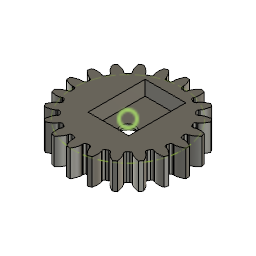
Servo_Gear (Autodesk Fusion 360 archive; units mm, degrees)
design "Servo_Gear"
description: Spur Gear; Module: 1.0; Num Teeth: 20; Pressure Angle: 20.0; Backlash: 0.00 mm
part number: 2026-08-10-18-01-22-383
Autodesk Fusion 360 part; units mm, degrees
(part 1 of 4)
sketch "Base Circle" plane through (0, 0, 0) normal (0, 0, 1) x (1, 0, 0)
  circle A0 centre (0, 0) radius 8.843
  circle A1 centre (0, 0) radius 2.6
  dimension "d9" = 5.2
  measures "d9" diameter of A1
extrude "Extrude1" add sketch "Base Circle" along normal blind 3.5
sketch "Gear Tooth" plane through (0, 0, 0) normal (0, 0, 1) x (1, 0, 0)
  spline S0 degree 5 poles (9.3559, -0.8768) (9.3606, -0.8772) (9.3699, -0.878) (9.3839, -0.8788) (9.4026, -0.8791) (9.426, -0.8785) (9.4495, -0.8772) (9.473, -0.8755) (9.4965, -0.8735) (9.52, -0.8714) (9.5435, -0.8691) (9.567, -0.8666) (9.5906, -0.8638) (9.6142, -0.8607) (9.6377, -0.8572) (9.6613, -0.8535) (9.6849, -0.8494) (9.7085, -0.8451) (9.7321, -0.8406) (9.7557, -0.836) (9.7793, -0.8311) (9.8029, -0.8261) (9.8265, -0.8208) (9.8501, -0.8153) (9.8737, -0.8096) (9.8973, -0.8037) (9.9209, -0.7977) (9.9445, -0.7914) (9.968, -0.7849) (9.9916, -0.7783) (10.0152, -0.7715) (10.0388, -0.7645) (10.0623, -0.7574) (10.0859, -0.7501) (10.1095, -0.7426) (10.133, -0.7349) (10.1565, -0.7271) (10.1801, -0.7191) (10.2036, -0.711) (10.2271, -0.7027) (10.2506, -0.6942) (10.2741, -0.6856) (10.2976, -0.6768) (10.321, -0.6679) (10.3445, -0.6588) (10.3679, -0.6496) (10.3913, -0.6402) (10.4148, -0.6307) (10.4382, -0.621) (10.4615, -0.6112) (10.4849, -0.6013) (10.5083, -0.5912) (10.5316, -0.5809) (10.5549, -0.5705) (10.5782, -0.56) (10.6015, -0.5493) (10.6248, -0.5385) (10.6481, -0.5276) (10.6713, -0.5165) (10.6945, -0.5053) (10.7177, -0.4939) (10.7409, -0.4824) (10.7641, -0.4708) (10.7872, -0.4591) (10.8103, -0.4472) (10.8334, -0.4352) (10.8565, -0.423) (10.8796, -0.4107) (10.9026, -0.3983) (10.9256, -0.3858) (10.9486, -0.3731) (10.967, -0.3629) (10.9807, -0.3552) (10.9899, -0.35) (10.9945, -0.3474) knots 0 0 0 0 0 0 0.01428571 0.02857143 0.04285714 0.05714286 0.07142857 0.08571429 0.1 0.11428571 0.12857143 0.14285714 0.15714286 0.17142857 0.18571429 0.2 0.21428571 0.22857143 0.24285714 0.25714286 0.27142857 0.28571429 0.3 0.31428571 0.32857143 0.34285714 0.35714286 0.37142857 0.38571429 0.4 0.41428571 0.42857143 0.44285714 0.45714286 0.47142857 0.48571429 0.5 0.51428571 0.52857143 0.54285714 0.55714286 0.57142857 0.58571429 0.6 0.61428571 0.62857143 0.64285714 0.65714286 0.67142857 0.68571429 0.7 0.71428571 0.72857143 0.74285714 0.75714286 0.77142857 0.78571429 0.8 0.81428571 0.82857143 0.84285714 0.85714286 0.87142857 0.88571429 0.9 0.91428571 0.92857143 0.94285714 0.95714286 0.97142857 0.98571429 1 1 1 1 1 1
  spline S1 degree 5 poles (9.3559, 0.8768) (9.3606, 0.8772) (9.3699, 0.878) (9.3839, 0.8788) (9.4026, 0.8791) (9.426, 0.8785) (9.4495, 0.8772) (9.473, 0.8755) (9.4965, 0.8735) (9.52, 0.8714) (9.5435, 0.8691) (9.567, 0.8666) (9.5906, 0.8638) (9.6142, 0.8607) (9.6377, 0.8572) (9.6613, 0.8535) (9.6849, 0.8494) (9.7085, 0.8451) (9.7321, 0.8406) (9.7557, 0.836) (9.7793, 0.8311) (9.8029, 0.8261) (9.8265, 0.8208) (9.8501, 0.8153) (9.8737, 0.8096) (9.8973, 0.8037) (9.9209, 0.7977) (9.9445, 0.7914) (9.968, 0.7849) (9.9916, 0.7783) (10.0152, 0.7715) (10.0388, 0.7645) (10.0623, 0.7574) (10.0859, 0.7501) (10.1095, 0.7426) (10.133, 0.7349) (10.1565, 0.7271) (10.1801, 0.7191) (10.2036, 0.711) (10.2271, 0.7027) (10.2506, 0.6942) (10.2741, 0.6856) (10.2976, 0.6768) (10.321, 0.6679) (10.3445, 0.6588) (10.3679, 0.6496) (10.3913, 0.6402) (10.4148, 0.6307) (10.4382, 0.621) (10.4615, 0.6112) (10.4849, 0.6013) (10.5083, 0.5912) (10.5316, 0.5809) (10.5549, 0.5705) (10.5782, 0.56) (10.6015, 0.5493) (10.6248, 0.5385) (10.6481, 0.5276) (10.6713, 0.5165) (10.6945, 0.5053) (10.7177, 0.4939) (10.7409, 0.4824) (10.7641, 0.4708) (10.7872, 0.4591) (10.8103, 0.4472) (10.8334, 0.4352) (10.8565, 0.423) (10.8796, 0.4107) (10.9026, 0.3983) (10.9256, 0.3858) (10.9486, 0.3731) (10.967, 0.3629) (10.9807, 0.3552) (10.9899, 0.35) (10.9945, 0.3474) knots 0 0 0 0 0 0 0.01428571 0.02857143 0.04285714 0.05714286 0.07142857 0.08571429 0.1 0.11428571 0.12857143 0.14285714 0.15714286 0.17142857 0.18571429 0.2 0.21428571 0.22857143 0.24285714 0.25714286 0.27142857 0.28571429 0.3 0.31428571 0.32857143 0.34285714 0.35714286 0.37142857 0.38571429 0.4 0.41428571 0.42857143 0.44285714 0.45714286 0.47142857 0.48571429 0.5 0.51428571 0.52857143 0.54285714 0.55714286 0.57142857 0.58571429 0.6 0.61428571 0.62857143 0.64285714 0.65714286 0.67142857 0.68571429 0.7 0.71428571 0.72857143 0.74285714 0.75714286 0.77142857 0.78571429 0.8 0.81428571 0.82857143 0.84285714 0.85714286 0.87142857 0.88571429 0.9 0.91428571 0.92857143 0.94285714 0.95714286 0.97142857 0.98571429 1 1 1 1 1 1
  arc A0 (10.9945, -0.3474) -> (10.9945, 0.3474) centre (0, 0) ccw
  line L0 (8.7945, -0.8242) -> (9.3559, -0.8768)
  line L1 (8.7945, 0.8242) -> (9.3559, 0.8768)
  line L2 (8.7945, -0.8242) -> (8.7945, 0.8242)
  point P0 (9.471, -0.8756)
  point P1 (9.5871, -0.8642)
  point P2 (9.7036, -0.846)
  point P3 (9.8206, -0.8221)
  point P4 (9.9379, -0.7931)
  point P5 (10.0553, -0.7595)
  point P6 (10.1729, -0.7215)
  point P7 (10.2906, -0.6794)
  point P8 (10.4082, -0.6333)
  point P9 (10.5258, -0.5834)
  point P10 (10.6433, -0.5298)
  point P11 (10.7606, -0.4725)
  point P12 (10.8777, -0.4117)
  point P13 (9.471, 0.8756)
  point P14 (9.5871, 0.8642)
  point P15 (9.7036, 0.846)
  point P16 (9.8206, 0.8221)
  point P17 (9.9379, 0.7931)
  point P18 (10.0553, 0.7595)
  point P19 (10.1729, 0.7215)
  point P20 (10.2906, 0.6794)
  point P21 (10.4082, 0.6333)
  point P22 (10.5258, 0.5834)
  point P23 (10.6433, 0.5298)
  point P24 (10.7606, 0.4725)
  point P25 (10.8777, 0.4117)
extrude "Extrude2" add sketch "Gear Tooth" along normal blind 3.5
fillet "Fillet1" radius 0.35 2 edges at (8.8044, -0.8251, 1.75) (8.8044, 0.8251, 1.75)
pattern_circular "C-Pattern1" count 20 over 360 about axis through (0, 0, 0) along (0, 0, 1) of "Extrude2", "Fillet1"
sketch "Diametrial Pitch Circle" plane through (0, 0, 0) normal (0, 0, 1) x (1, 0, 0)
  circle A0 centre (0, 0) radius 10 construction
extrude "Extrude3" add 1 faces at (6.7196, 0, 3.5) along direction (0, 0, 1) blind 0.4
sketch "Sketch4" plane through (0, 0, 3.9) normal (0, 0, 1) x (-1, 0, 0)
  arc A0 (-8.6959, 1.6061) -> (-8.7666, 1.1597) centre (0, 0) ccw
  arc A1 (-9.1463, 0.8572) -> (-8.7666, 1.1597) centre (-9.1136, 1.2056) ccw
  line L0 (-9.1463, 0.8572) -> (-9.3559, 0.8768)
  spline S0 degree 5 poles (-9.3559, 0.8768) (-9.3606, 0.8772) (-9.3699, 0.878) (-9.3839, 0.8788) (-9.4026, 0.8791) (-9.426, 0.8785) (-9.4495, 0.8772) (-9.473, 0.8755) (-9.4965, 0.8735) (-9.52, 0.8714) (-9.5435, 0.8691) (-9.567, 0.8666) (-9.5906, 0.8638) (-9.6142, 0.8607) (-9.6377, 0.8572) (-9.6613, 0.8535) (-9.6849, 0.8494) (-9.7085, 0.8451) (-9.7321, 0.8406) (-9.7557, 0.836) (-9.7793, 0.8311) (-9.8029, 0.8261) (-9.8265, 0.8208) (-9.8501, 0.8153) (-9.8737, 0.8096) (-9.8973, 0.8037) (-9.9209, 0.7977) (-9.9445, 0.7914) (-9.968, 0.7849) (-9.9916, 0.7783) (-10.0152, 0.7715) (-10.0388, 0.7645) (-10.0623, 0.7574) (-10.0859, 0.7501) (-10.1095, 0.7426) (-10.133, 0.7349) (-10.1565, 0.7271) (-10.1801, 0.7191) (-10.2036, 0.711) (-10.2271, 0.7027) (-10.2506, 0.6942) (-10.2741, 0.6856) (-10.2976, 0.6768) (-10.321, 0.6679) (-10.3445, 0.6588) (-10.3679, 0.6496) (-10.3913, 0.6402) (-10.4148, 0.6307) (-10.4382, 0.621) (-10.4615, 0.6112) (-10.4849, 0.6013) (-10.5083, 0.5912) (-10.5316, 0.5809) (-10.5549, 0.5705) (-10.5782, 0.56) (-10.6015, 0.5493) (-10.6248, 0.5385) (-10.6481, 0.5276) (-10.6713, 0.5165) (-10.6945, 0.5053) (-10.7177, 0.4939) (-10.7409, 0.4824) (-10.7641, 0.4708) (-10.7872, 0.4591) (-10.8103, 0.4472) (-10.8334, 0.4352) (-10.8565, 0.423) (-10.8796, 0.4107) (-10.9026, 0.3983) (-10.9256, 0.3858) (-10.9486, 0.3731) (-10.967, 0.3629) (-10.9807, 0.3552) (-10.9899, 0.35) (-10.9945, 0.3474) knots 0 0 0 0 0 0 0.01428571 0.02857143 0.04285714 0.05714286 0.07142857 0.08571429 0.1 0.11428571 0.12857143 0.14285714 0.15714286 0.17142857 0.18571429 0.2 0.21428571 0.22857143 0.24285714 0.25714286 0.27142857 0.28571429 0.3 0.31428571 0.32857143 0.34285714 0.35714286 0.37142857 0.38571429 0.4 0.41428571 0.42857143 0.44285714 0.45714286 0.47142857 0.48571429 0.5 0.51428571 0.52857143 0.54285714 0.55714286 0.57142857 0.58571429 0.6 0.61428571 0.62857143 0.64285714 0.65714286 0.67142857 0.68571429 0.7 0.71428571 0.72857143 0.74285714 0.75714286 0.77142857 0.78571429 0.8 0.81428571 0.82857143 0.84285714 0.85714286 0.87142857 0.88571429 0.9 0.91428571 0.92857143 0.94285714 0.95714286 0.97142857 0.98571429 1 1 1 1 1 1
  arc A2 (-10.9945, 0.3474) -> (-10.9945, -0.3474) centre (0, 0) ccw
  spline S1 degree 5 poles (-10.9945, -0.3474) (-10.9899, -0.35) (-10.9807, -0.3552) (-10.967, -0.3629) (-10.9486, -0.3731) (-10.9256, -0.3858) (-10.9026, -0.3983) (-10.8796, -0.4107) (-10.8565, -0.423) (-10.8334, -0.4352) (-10.8103, -0.4472) (-10.7872, -0.4591) (-10.7641, -0.4708) (-10.7409, -0.4824) (-10.7177, -0.4939) (-10.6945, -0.5053) (-10.6713, -0.5165) (-10.6481, -0.5276) (-10.6248, -0.5385) (-10.6015, -0.5493) (-10.5782, -0.56) (-10.5549, -0.5705) (-10.5316, -0.5809) (-10.5083, -0.5912) (-10.4849, -0.6013) (-10.4615, -0.6112) (-10.4382, -0.621) (-10.4148, -0.6307) (-10.3913, -0.6402) (-10.3679, -0.6496) (-10.3445, -0.6588) (-10.321, -0.6679) (-10.2976, -0.6768) (-10.2741, -0.6856) (-10.2506, -0.6942) (-10.2271, -0.7027) (-10.2036, -0.711) (-10.1801, -0.7191) (-10.1565, -0.7271) (-10.133, -0.7349) (-10.1095, -0.7426) (-10.0859, -0.7501) (-10.0623, -0.7574) (-10.0388, -0.7645) (-10.0152, -0.7715) (-9.9916, -0.7783) (-9.968, -0.7849) (-9.9445, -0.7914) (-9.9209, -0.7977) (-9.8973, -0.8037) (-9.8737, -0.8096) (-9.8501, -0.8153) (-9.8265, -0.8208) (-9.8029, -0.8261) (-9.7793, -0.8311) (-9.7557, -0.836) (-9.7321, -0.8406) (-9.7085, -0.8451) (-9.6849, -0.8494) (-9.6613, -0.8535) (-9.6377, -0.8572) (-9.6142, -0.8607) (-9.5906, -0.8638) (-9.567, -0.8666) (-9.5435, -0.8691) (-9.52, -0.8714) (-9.4965, -0.8735) (-9.473, -0.8755) (-9.4495, -0.8772) (-9.426, -0.8785) (-9.4026, -0.8791) (-9.3839, -0.8788) (-9.3699, -0.878) (-9.3606, -0.8772) (-9.3559, -0.8768) knots -1 -1 -1 -1 -1 -1 -0.98571429 -0.97142857 -0.95714286 -0.94285714 -0.92857143 -0.91428571 -0.9 -0.88571429 -0.87142857 -0.85714286 -0.84285714 -0.82857143 -0.81428571 -0.8 -0.78571429 -0.77142857 -0.75714286 -0.74285714 -0.72857143 -0.71428571 -0.7 -0.68571429 -0.67142857 -0.65714286 -0.64285714 -0.62857143 -0.61428571 -0.6 -0.58571429 -0.57142857 -0.55714286 -0.54285714 -0.52857143 -0.51428571 -0.5 -0.48571429 -0.47142857 -0.45714286 -0.44285714 -0.42857143 -0.41428571 -0.4 -0.38571429 -0.37142857 -0.35714286 -0.34285714 -0.32857143 -0.31428571 -0.3 -0.28571429 -0.27142857 -0.25714286 -0.24285714 -0.22857143 -0.21428571 -0.2 -0.18571429 -0.17142857 -0.15714286 -0.14285714 -0.12857143 -0.11428571 -0.1 -0.08571429 -0.07142857 -0.05714286 -0.04285714 -0.02857143 -0.01428571 0 0 0 0 0 0
  line L1 (-9.3559, -0.8768) -> (-9.1463, -0.8572)
  arc A3 (-8.7666, -1.1597) -> (-9.1463, -0.8572) centre (-9.1136, -1.2056) ccw
  arc A4 (-8.7666, -1.1597) -> (-8.6959, -1.6061) centre (0, 0) ccw
  arc A5 (-8.9635, -2.0111) -> (-8.6959, -1.6061) centre (-9.0401, -1.6696) ccw
  line L2 (-8.9635, -2.0111) -> (-9.169, -2.0572)
  spline S2 degree 5 poles (-9.169, -2.0572) (-9.1735, -2.0583) (-9.1826, -2.0604) (-9.1962, -2.064) (-9.2141, -2.0695) (-9.2361, -2.0773) (-9.2581, -2.0858) (-9.2799, -2.0947) (-9.3016, -2.1038) (-9.3233, -2.1131) (-9.345, -2.1225) (-9.3666, -2.1322) (-9.3881, -2.1421) (-9.4096, -2.1524) (-9.4309, -2.1629) (-9.4522, -2.1738) (-9.4734, -2.185) (-9.4945, -2.1963) (-9.5155, -2.2079) (-9.5365, -2.2196) (-9.5575, -2.2315) (-9.5784, -2.2436) (-9.5992, -2.2559) (-9.6199, -2.2684) (-9.6406, -2.2811) (-9.6612, -2.294) (-9.6818, -2.3071) (-9.7023, -2.3204) (-9.7227, -2.3338) (-9.7431, -2.3474) (-9.7634, -2.3611) (-9.7837, -2.375) (-9.8039, -2.3891) (-9.8241, -2.4033) (-9.8441, -2.4177) (-9.8642, -2.4323) (-9.8841, -2.447) (-9.904, -2.4619) (-9.9239, -2.4769) (-9.9437, -2.492) (-9.9634, -2.5074) (-9.9831, -2.5228) (-10.0027, -2.5384) (-10.0223, -2.5541) (-10.0418, -2.57) (-10.0612, -2.586) (-10.0806, -2.6022) (-10.0999, -2.6185) (-10.1192, -2.6349) (-10.1384, -2.6515) (-10.1575, -2.6682) (-10.1766, -2.685) (-10.1957, -2.702) (-10.2146, -2.719) (-10.2335, -2.7363) (-10.2524, -2.7536) (-10.2712, -2.7711) (-10.2899, -2.7887) (-10.3086, -2.8064) (-10.3272, -2.8242) (-10.3458, -2.8422) (-10.3643, -2.8603) (-10.3827, -2.8785) (-10.4011, -2.8968) (-10.4194, -2.9153) (-10.4377, -2.9339) (-10.4559, -2.9525) (-10.474, -2.9713) (-10.4921, -2.9903) (-10.5101, -3.0093) (-10.528, -3.0284) (-10.5424, -3.0439) (-10.5531, -3.0555) (-10.5602, -3.0632) (-10.5638, -3.0671) knots 0 0 0 0 0 0 0.01428571 0.02857143 0.04285714 0.05714286 0.07142857 0.08571429 0.1 0.11428571 0.12857143 0.14285714 0.15714286 0.17142857 0.18571429 0.2 0.21428571 0.22857143 0.24285714 0.25714286 0.27142857 0.28571429 0.3 0.31428571 0.32857143 0.34285714 0.35714286 0.37142857 0.38571429 0.4 0.41428571 0.42857143 0.44285714 0.45714286 0.47142857 0.48571429 0.5 0.51428571 0.52857143 0.54285714 0.55714286 0.57142857 0.58571429 0.6 0.61428571 0.62857143 0.64285714 0.65714286 0.67142857 0.68571429 0.7 0.71428571 0.72857143 0.74285714 0.75714286 0.77142857 0.78571429 0.8 0.81428571 0.82857143 0.84285714 0.85714286 0.87142857 0.88571429 0.9 0.91428571 0.92857143 0.94285714 0.95714286 0.97142857 0.98571429 1 1 1 1 1 1
  arc A6 (-10.5638, -3.0671) -> (-10.3491, -3.7279) centre (0, 0) ccw
  spline S3 degree 5 poles (-10.3491, -3.7279) (-10.3439, -3.7289) (-10.3336, -3.731) (-10.3181, -3.7341) (-10.2974, -3.7382) (-10.2717, -3.7431) (-10.2459, -3.7479) (-10.2202, -3.7526) (-10.1944, -3.7572) (-10.1687, -3.7616) (-10.143, -3.7659) (-10.1174, -3.77) (-10.0917, -3.774) (-10.0661, -3.7779) (-10.0405, -3.7817) (-10.0149, -3.7853) (-9.9894, -3.7888) (-9.9639, -3.7922) (-9.9384, -3.7954) (-9.9129, -3.7985) (-9.8875, -3.8014) (-9.862, -3.8043) (-9.8366, -3.8069) (-9.8113, -3.8095) (-9.7859, -3.8119) (-9.7606, -3.8141) (-9.7354, -3.8162) (-9.7101, -3.8182) (-9.6849, -3.82) (-9.6597, -3.8217) (-9.6346, -3.8232) (-9.6095, -3.8246) (-9.5844, -3.8258) (-9.5594, -3.8269) (-9.5344, -3.8279) (-9.5094, -3.8286) (-9.4845, -3.8293) (-9.4596, -3.8298) (-9.4347, -3.8301) (-9.4099, -3.8302) (-9.3852, -3.8302) (-9.3605, -3.8301) (-9.3358, -3.8298) (-9.3112, -3.8293) (-9.2866, -3.8286) (-9.2621, -3.8278) (-9.2376, -3.8268) (-9.2132, -3.8257) (-9.1888, -3.8243) (-9.1645, -3.8228) (-9.1402, -3.8211) (-9.116, -3.8193) (-9.0919, -3.8172) (-9.0678, -3.8149) (-9.0438, -3.8124) (-9.0199, -3.8097) (-8.996, -3.8069) (-8.9722, -3.8038) (-8.9484, -3.8006) (-8.9247, -3.7972) (-8.9011, -3.7935) (-8.8776, -3.7895) (-8.8543, -3.7852) (-8.831, -3.7806) (-8.8078, -3.7757) (-8.7848, -3.7706) (-8.7617, -3.7653) (-8.7388, -3.7599) (-8.7159, -3.7543) (-8.6932, -3.7483) (-8.6708, -3.7416) (-8.6531, -3.7355) (-8.64, -3.7305) (-8.6314, -3.7269) (-8.6271, -3.725) knots -1 -1 -1 -1 -1 -1 -0.98571429 -0.97142857 -0.95714286 -0.94285714 -0.92857143 -0.91428571 -0.9 -0.88571429 -0.87142857 -0.85714286 -0.84285714 -0.82857143 -0.81428571 -0.8 -0.78571429 -0.77142857 -0.75714286 -0.74285714 -0.72857143 -0.71428571 -0.7 -0.68571429 -0.67142857 -0.65714286 -0.64285714 -0.62857143 -0.61428571 -0.6 -0.58571429 -0.57142857 -0.55714286 -0.54285714 -0.52857143 -0.51428571 -0.5 -0.48571429 -0.47142857 -0.45714286 -0.44285714 -0.42857143 -0.41428571 -0.4 -0.38571429 -0.37142857 -0.35714286 -0.34285714 -0.32857143 -0.31428571 -0.3 -0.28571429 -0.27142857 -0.25714286 -0.24285714 -0.22857143 -0.21428571 -0.2 -0.18571429 -0.17142857 -0.15714286 -0.14285714 -0.12857143 -0.11428571 -0.1 -0.08571429 -0.07142857 -0.05714286 -0.04285714 -0.02857143 -0.01428571 0 0 0 0 0 0
  line L3 (-8.6271, -3.725) -> (-8.4337, -3.6416)
  arc A7 (-7.9792, -3.812) -> (-8.4337, -3.6416) centre (-8.295, -3.9629) ccw
  arc A8 (-7.9792, -3.812) -> (-7.774, -4.2146) centre (0, 0) ccw
  arc A9 (-7.9033, -4.6826) -> (-7.774, -4.2146) centre (-8.0817, -4.3815) ccw
  line L4 (-7.9033, -4.6826) -> (-8.0845, -4.7899)
  spline S4 degree 5 poles (-8.0845, -4.7899) (-8.0885, -4.7923) (-8.0965, -4.7972) (-8.1083, -4.8048) (-8.1236, -4.8155) (-8.1422, -4.8298) (-8.1604, -4.8446) (-8.1784, -4.8598) (-8.1962, -4.8752) (-8.214, -4.8907) (-8.2317, -4.9064) (-8.2493, -4.9223) (-8.2667, -4.9384) (-8.2839, -4.9547) (-8.301, -4.9714) (-8.3178, -4.9883) (-8.3345, -5.0055) (-8.3511, -5.0228) (-8.3675, -5.0403) (-8.3839, -5.0579) (-8.4001, -5.0757) (-8.4162, -5.0937) (-8.4322, -5.1118) (-8.4481, -5.1301) (-8.4639, -5.1486) (-8.4795, -5.1672) (-8.495, -5.186) (-8.5104, -5.205) (-8.5257, -5.224) (-8.5409, -5.2433) (-8.556, -5.2626) (-8.5709, -5.2821) (-8.5858, -5.3017) (-8.6006, -5.3215) (-8.6152, -5.3414) (-8.6298, -5.3614) (-8.6442, -5.3816) (-8.6585, -5.4019) (-8.6728, -5.4223) (-8.6869, -5.4428) (-8.701, -5.4635) (-8.7149, -5.4843) (-8.7287, -5.5052) (-8.7425, -5.5262) (-8.7561, -5.5473) (-8.7697, -5.5686) (-8.7831, -5.5899) (-8.7964, -5.6114) (-8.8097, -5.633) (-8.8228, -5.6546) (-8.8359, -5.6764) (-8.8488, -5.6983) (-8.8617, -5.7204) (-8.8745, -5.7425) (-8.8871, -5.7647) (-8.8997, -5.787) (-8.9122, -5.8094) (-8.9246, -5.832) (-8.9368, -5.8546) (-8.949, -5.8773) (-8.9611, -5.9001) (-8.9731, -5.923) (-8.985, -5.9461) (-8.9969, -5.9692) (-9.0086, -5.9924) (-9.0202, -6.0157) (-9.0317, -6.0391) (-9.0432, -6.0626) (-9.0545, -6.0861) (-9.0658, -6.1098) (-9.0769, -6.1336) (-9.0858, -6.1526) (-9.0924, -6.167) (-9.0967, -6.1766) (-9.0989, -6.1814) knots 0 0 0 0 0 0 0.01428571 0.02857143 0.04285714 0.05714286 0.07142857 0.08571429 0.1 0.11428571 0.12857143 0.14285714 0.15714286 0.17142857 0.18571429 0.2 0.21428571 0.22857143 0.24285714 0.25714286 0.27142857 0.28571429 0.3 0.31428571 0.32857143 0.34285714 0.35714286 0.37142857 0.38571429 0.4 0.41428571 0.42857143 0.44285714 0.45714286 0.47142857 0.48571429 0.5 0.51428571 0.52857143 0.54285714 0.55714286 0.57142857 0.58571429 0.6 0.61428571 0.62857143 0.64285714 0.65714286 0.67142857 0.68571429 0.7 0.71428571 0.72857143 0.74285714 0.75714286 0.77142857 0.78571429 0.8 0.81428571 0.82857143 0.84285714 0.85714286 0.87142857 0.88571429 0.9 0.91428571 0.92857143 0.94285714 0.95714286 0.97142857 0.98571429 1 1 1 1 1 1
  arc A10 (-9.0989, -6.1814) -> (-8.6906, -6.7435) centre (0, 0) ccw
  spline S5 degree 5 poles (-8.6906, -6.7435) (-8.6853, -6.7429) (-8.6749, -6.7417) (-8.6592, -6.7398) (-8.6383, -6.7373) (-8.6122, -6.734) (-8.5863, -6.7306) (-8.5603, -6.7271) (-8.5345, -6.7235) (-8.5086, -6.7198) (-8.4829, -6.7159) (-8.4572, -6.7119) (-8.4316, -6.7079) (-8.406, -6.7036) (-8.3805, -6.6993) (-8.355, -6.6949) (-8.3297, -6.6903) (-8.3044, -6.6856) (-8.2791, -6.6808) (-8.2539, -6.6758) (-8.2288, -6.6708) (-8.2038, -6.6656) (-8.1788, -6.6603) (-8.1539, -6.6549) (-8.1291, -6.6493) (-8.1043, -6.6436) (-8.0796, -6.6378) (-8.055, -6.6319) (-8.0304, -6.6258) (-8.006, -6.6197) (-7.9816, -6.6133) (-7.9573, -6.6069) (-7.9331, -6.6003) (-7.9089, -6.5936) (-7.8848, -6.5868) (-7.8609, -6.5798) (-7.837, -6.5727) (-7.8131, -6.5655) (-7.7894, -6.5581) (-7.7658, -6.5506) (-7.7422, -6.543) (-7.7188, -6.5352) (-7.6954, -6.5273) (-7.6722, -6.5192) (-7.649, -6.511) (-7.6259, -6.5026) (-7.6029, -6.4941) (-7.5801, -6.4855) (-7.5573, -6.4767) (-7.5346, -6.4677) (-7.5121, -6.4586) (-7.4897, -6.4493) (-7.4673, -6.4399) (-7.4452, -6.4303) (-7.4231, -6.4205) (-7.4011, -6.4106) (-7.3793, -6.4005) (-7.3576, -6.3902) (-7.336, -6.3798) (-7.3145, -6.3692) (-7.2932, -6.3584) (-7.2721, -6.3474) (-7.2512, -6.3361) (-7.2305, -6.3245) (-7.21, -6.3126) (-7.1896, -6.3007) (-7.1694, -6.2886) (-7.1492, -6.2763) (-7.1292, -6.2639) (-7.1095, -6.2512) (-7.0902, -6.2379) (-7.0752, -6.2267) (-7.0643, -6.2178) (-7.0572, -6.2117) (-7.0537, -6.2086) knots -1 -1 -1 -1 -1 -1 -0.98571429 -0.97142857 -0.95714286 -0.94285714 -0.92857143 -0.91428571 -0.9 -0.88571429 -0.87142857 -0.85714286 -0.84285714 -0.82857143 -0.81428571 -0.8 -0.78571429 -0.77142857 -0.75714286 -0.74285714 -0.72857143 -0.71428571 -0.7 -0.68571429 -0.67142857 -0.65714286 -0.64285714 -0.62857143 -0.61428571 -0.6 -0.58571429 -0.57142857 -0.55714286 -0.54285714 -0.52857143 -0.51428571 -0.5 -0.48571429 -0.47142857 -0.45714286 -0.44285714 -0.42857143 -0.41428571 -0.4 -0.38571429 -0.37142857 -0.35714286 -0.34285714 -0.32857143 -0.31428571 -0.3 -0.28571429 -0.27142857 -0.25714286 -0.24285714 -0.22857143 -0.21428571 -0.2 -0.18571429 -0.17142857 -0.15714286 -0.14285714 -0.12857143 -0.11428571 -0.1 -0.08571429 -0.07142857 -0.05714286 -0.04285714 -0.02857143 -0.01428571 0 0 0 0 0 0
  line L5 (-7.0537, -6.2086) -> (-6.8957, -6.0695)
  arc A11 (-6.4107, -6.0911) -> (-6.8957, -6.0695) centre (-6.6644, -6.3322) ccw
  arc A12 (-6.4107, -6.0911) -> (-6.0911, -6.4107) centre (0, 0) ccw
  arc A13 (-6.0695, -6.8957) -> (-6.0911, -6.4107) centre (-6.3322, -6.6644) ccw
  line L6 (-6.0695, -6.8957) -> (-6.2086, -7.0537)
  spline S6 degree 5 poles (-6.2086, -7.0537) (-6.2117, -7.0572) (-6.2178, -7.0643) (-6.2267, -7.0752) (-6.2379, -7.0902) (-6.2512, -7.1095) (-6.2639, -7.1292) (-6.2763, -7.1492) (-6.2886, -7.1694) (-6.3007, -7.1896) (-6.3126, -7.21) (-6.3245, -7.2305) (-6.3361, -7.2512) (-6.3474, -7.2721) (-6.3584, -7.2932) (-6.3692, -7.3145) (-6.3798, -7.336) (-6.3902, -7.3576) (-6.4005, -7.3793) (-6.4106, -7.4011) (-6.4205, -7.4231) (-6.4303, -7.4452) (-6.4399, -7.4673) (-6.4493, -7.4897) (-6.4586, -7.5121) (-6.4677, -7.5346) (-6.4767, -7.5573) (-6.4855, -7.5801) (-6.4941, -7.6029) (-6.5026, -7.6259) (-6.511, -7.649) (-6.5192, -7.6722) (-6.5273, -7.6954) (-6.5352, -7.7188) (-6.543, -7.7422) (-6.5506, -7.7658) (-6.5581, -7.7894) (-6.5655, -7.8131) (-6.5727, -7.837) (-6.5798, -7.8609) (-6.5868, -7.8848) (-6.5936, -7.9089) (-6.6003, -7.9331) (-6.6069, -7.9573) (-6.6133, -7.9816) (-6.6197, -8.006) (-6.6258, -8.0304) (-6.6319, -8.055) (-6.6378, -8.0796) (-6.6436, -8.1043) (-6.6493, -8.1291) (-6.6549, -8.1539) (-6.6603, -8.1788) (-6.6656, -8.2038) (-6.6708, -8.2288) (-6.6758, -8.2539) (-6.6808, -8.2791) (-6.6856, -8.3044) (-6.6903, -8.3297) (-6.6949, -8.355) (-6.6993, -8.3805) (-6.7036, -8.406) (-6.7079, -8.4316) (-6.7119, -8.4572) (-6.7159, -8.4829) (-6.7198, -8.5086) (-6.7235, -8.5345) (-6.7271, -8.5603) (-6.7306, -8.5863) (-6.734, -8.6122) (-6.7373, -8.6383) (-6.7398, -8.6592) (-6.7417, -8.6749) (-6.7429, -8.6853) (-6.7435, -8.6906) knots 0 0 0 0 0 0 0.01428571 0.02857143 0.04285714 0.05714286 0.07142857 0.08571429 0.1 0.11428571 0.12857143 0.14285714 0.15714286 0.17142857 0.18571429 0.2 0.21428571 0.22857143 0.24285714 0.25714286 0.27142857 0.28571429 0.3 0.31428571 0.32857143 0.34285714 0.35714286 0.37142857 0.38571429 0.4 0.41428571 0.42857143 0.44285714 0.45714286 0.47142857 0.48571429 0.5 0.51428571 0.52857143 0.54285714 0.55714286 0.57142857 0.58571429 0.6 0.61428571 0.62857143 0.64285714 0.65714286 0.67142857 0.68571429 0.7 0.71428571 0.72857143 0.74285714 0.75714286 0.77142857 0.78571429 0.8 0.81428571 0.82857143 0.84285714 0.85714286 0.87142857 0.88571429 0.9 0.91428571 0.92857143 0.94285714 0.95714286 0.97142857 0.98571429 1 1 1 1 1 1
  arc A14 (-6.7435, -8.6906) -> (-6.1814, -9.0989) centre (0, 0) ccw
  spline S7 degree 5 poles (-6.1814, -9.0989) (-6.1766, -9.0967) (-6.167, -9.0924) (-6.1526, -9.0858) (-6.1336, -9.0769) (-6.1098, -9.0658) (-6.0861, -9.0545) (-6.0626, -9.0432) (-6.0391, -9.0317) (-6.0157, -9.0202) (-5.9924, -9.0086) (-5.9692, -8.9969) (-5.9461, -8.985) (-5.923, -8.9731) (-5.9001, -8.9611) (-5.8773, -8.949) (-5.8546, -8.9368) (-5.832, -8.9246) (-5.8094, -8.9122) (-5.787, -8.8997) (-5.7647, -8.8871) (-5.7425, -8.8745) (-5.7204, -8.8617) (-5.6983, -8.8488) (-5.6764, -8.8359) (-5.6546, -8.8228) (-5.633, -8.8097) (-5.6114, -8.7964) (-5.5899, -8.7831) (-5.5686, -8.7697) (-5.5473, -8.7561) (-5.5262, -8.7425) (-5.5052, -8.7287) (-5.4843, -8.7149) (-5.4635, -8.701) (-5.4428, -8.6869) (-5.4223, -8.6728) (-5.4019, -8.6585) (-5.3816, -8.6442) (-5.3614, -8.6298) (-5.3414, -8.6152) (-5.3215, -8.6006) (-5.3017, -8.5858) (-5.2821, -8.5709) (-5.2626, -8.556) (-5.2433, -8.5409) (-5.224, -8.5257) (-5.205, -8.5104) (-5.186, -8.495) (-5.1672, -8.4795) (-5.1486, -8.4639) (-5.1301, -8.4481) (-5.1118, -8.4322) (-5.0937, -8.4162) (-5.0757, -8.4001) (-5.0579, -8.3839) (-5.0403, -8.3675) (-5.0228, -8.3511) (-5.0055, -8.3345) (-4.9883, -8.3178) (-4.9714, -8.301) (-4.9547, -8.2839) (-4.9384, -8.2667) (-4.9223, -8.2493) (-4.9064, -8.2317) (-4.8907, -8.214) (-4.8752, -8.1962) (-4.8598, -8.1784) (-4.8446, -8.1604) (-4.8298, -8.1422) (-4.8155, -8.1236) (-4.8048, -8.1083) (-4.7972, -8.0965) (-4.7923, -8.0885) (-4.7899, -8.0845) knots -1 -1 -1 -1 -1 -1 -0.98571429 -0.97142857 -0.95714286 -0.94285714 -0.92857143 -0.91428571 -0.9 -0.88571429 -0.87142857 -0.85714286 -0.84285714 -0.82857143 -0.81428571 -0.8 -0.78571429 -0.77142857 -0.75714286 -0.74285714 -0.72857143 -0.71428571 -0.7 -0.68571429 -0.67142857 -0.65714286 -0.64285714 -0.62857143 -0.61428571 -0.6 -0.58571429 -0.57142857 -0.55714286 -0.54285714 -0.52857143 -0.51428571 -0.5 -0.48571429 -0.47142857 -0.45714286 -0.44285714 -0.42857143 -0.41428571 -0.4 -0.38571429 -0.37142857 -0.35714286 -0.34285714 -0.32857143 -0.31428571 -0.3 -0.28571429 -0.27142857 -0.25714286 -0.24285714 -0.22857143 -0.21428571 -0.2 -0.18571429 -0.17142857 -0.15714286 -0.14285714 -0.12857143 -0.11428571 -0.1 -0.08571429 -0.07142857 -0.05714286 -0.04285714 -0.02857143 -0.01428571 0 0 0 0 0 0
  line L7 (-4.7899, -8.0845) -> (-4.6826, -7.9033)
  arc A15 (-4.2146, -7.774) -> (-4.6826, -7.9033) centre (-4.3815, -8.0817) ccw
  arc A16 (-4.2146, -7.774) -> (-3.812, -7.9792) centre (0, 0) ccw
  arc A17 (-3.6416, -8.4337) -> (-3.812, -7.9792) centre (-3.9629, -8.295) ccw
  line L8 (-3.6416, -8.4337) -> (-3.725, -8.6271)
  spline S8 degree 5 poles (-3.725, -8.6271) (-3.7269, -8.6314) (-3.7305, -8.64) (-3.7355, -8.6531) (-3.7416, -8.6708) (-3.7483, -8.6932) (-3.7543, -8.7159) (-3.7599, -8.7388) (-3.7653, -8.7617) (-3.7706, -8.7848) (-3.7757, -8.8078) (-3.7806, -8.831) (-3.7852, -8.8543) (-3.7895, -8.8776) (-3.7935, -8.9011) (-3.7972, -8.9247) (-3.8006, -8.9484) (-3.8038, -8.9722) (-3.8069, -8.996) (-3.8097, -9.0199) (-3.8124, -9.0438) (-3.8149, -9.0678) (-3.8172, -9.0919) (-3.8193, -9.116) (-3.8211, -9.1402) (-3.8228, -9.1645) (-3.8243, -9.1888) (-3.8257, -9.2132) (-3.8268, -9.2376) (-3.8278, -9.2621) (-3.8286, -9.2866) (-3.8293, -9.3112) (-3.8298, -9.3358) (-3.8301, -9.3605) (-3.8302, -9.3852) (-3.8302, -9.4099) (-3.8301, -9.4347) (-3.8298, -9.4596) (-3.8293, -9.4845) (-3.8286, -9.5094) (-3.8279, -9.5344) (-3.8269, -9.5594) (-3.8258, -9.5844) (-3.8246, -9.6095) (-3.8232, -9.6346) (-3.8217, -9.6597) (-3.82, -9.6849) (-3.8182, -9.7101) (-3.8162, -9.7354) (-3.8141, -9.7606) (-3.8119, -9.7859) (-3.8095, -9.8113) (-3.8069, -9.8366) (-3.8043, -9.862) (-3.8014, -9.8875) (-3.7985, -9.9129) (-3.7954, -9.9384) (-3.7922, -9.9639) (-3.7888, -9.9894) (-3.7853, -10.0149) (-3.7817, -10.0405) (-3.7779, -10.0661) (-3.774, -10.0917) (-3.77, -10.1174) (-3.7659, -10.143) (-3.7616, -10.1687) (-3.7572, -10.1944) (-3.7526, -10.2202) (-3.7479, -10.2459) (-3.7431, -10.2717) (-3.7382, -10.2974) (-3.7341, -10.3181) (-3.731, -10.3336) (-3.7289, -10.3439) (-3.7279, -10.3491) knots 0 0 0 0 0 0 0.01428571 0.02857143 0.04285714 0.05714286 0.07142857 0.08571429 0.1 0.11428571 0.12857143 0.14285714 0.15714286 0.17142857 0.18571429 0.2 0.21428571 0.22857143 0.24285714 0.25714286 0.27142857 0.28571429 0.3 0.31428571 0.32857143 0.34285714 0.35714286 0.37142857 0.38571429 0.4 0.41428571 0.42857143 0.44285714 0.45714286 0.47142857 0.48571429 0.5 0.51428571 0.52857143 0.54285714 0.55714286 0.57142857 0.58571429 0.6 0.61428571 0.62857143 0.64285714 0.65714286 0.67142857 0.68571429 0.7 0.71428571 0.72857143 0.74285714 0.75714286 0.77142857 0.78571429 0.8 0.81428571 0.82857143 0.84285714 0.85714286 0.87142857 0.88571429 0.9 0.91428571 0.92857143 0.94285714 0.95714286 0.97142857 0.98571429 1 1 1 1 1 1
  arc A18 (-3.7279, -10.3491) -> (-3.0671, -10.5638) centre (0, 0) ccw
  spline S9 degree 5 poles (-3.0671, -10.5638) (-3.0632, -10.5602) (-3.0555, -10.5531) (-3.0439, -10.5424) (-3.0284, -10.528) (-3.0093, -10.5101) (-2.9903, -10.4921) (-2.9713, -10.474) (-2.9525, -10.4559) (-2.9339, -10.4377) (-2.9153, -10.4194) (-2.8968, -10.4011) (-2.8785, -10.3827) (-2.8603, -10.3643) (-2.8422, -10.3458) (-2.8242, -10.3272) (-2.8064, -10.3086) (-2.7887, -10.2899) (-2.7711, -10.2712) (-2.7536, -10.2524) (-2.7363, -10.2335) (-2.719, -10.2146) (-2.702, -10.1957) (-2.685, -10.1766) (-2.6682, -10.1575) (-2.6515, -10.1384) (-2.6349, -10.1192) (-2.6185, -10.0999) (-2.6022, -10.0806) (-2.586, -10.0612) (-2.57, -10.0418) (-2.5541, -10.0223) (-2.5384, -10.0027) (-2.5228, -9.9831) (-2.5074, -9.9634) (-2.492, -9.9437) (-2.4769, -9.9239) (-2.4619, -9.904) (-2.447, -9.8841) (-2.4323, -9.8642) (-2.4177, -9.8441) (-2.4033, -9.8241) (-2.3891, -9.8039) (-2.375, -9.7837) (-2.3611, -9.7634) (-2.3474, -9.7431) (-2.3338, -9.7227) (-2.3204, -9.7023) (-2.3071, -9.6818) (-2.294, -9.6612) (-2.2811, -9.6406) (-2.2684, -9.6199) (-2.2559, -9.5992) (-2.2436, -9.5784) (-2.2315, -9.5575) (-2.2196, -9.5365) (-2.2079, -9.5155) (-2.1963, -9.4945) (-2.185, -9.4734) (-2.1738, -9.4522) (-2.1629, -9.4309) (-2.1524, -9.4096) (-2.1421, -9.3881) (-2.1322, -9.3666) (-2.1225, -9.345) (-2.1131, -9.3233) (-2.1038, -9.3016) (-2.0947, -9.2799) (-2.0858, -9.2581) (-2.0773, -9.2361) (-2.0695, -9.2141) (-2.064, -9.1962) (-2.0604, -9.1826) (-2.0583, -9.1735) (-2.0572, -9.169) knots -1 -1 -1 -1 -1 -1 -0.98571429 -0.97142857 -0.95714286 -0.94285714 -0.92857143 -0.91428571 -0.9 -0.88571429 -0.87142857 -0.85714286 -0.84285714 -0.82857143 -0.81428571 -0.8 -0.78571429 -0.77142857 -0.75714286 -0.74285714 -0.72857143 -0.71428571 -0.7 -0.68571429 -0.67142857 -0.65714286 -0.64285714 -0.62857143 -0.61428571 -0.6 -0.58571429 -0.57142857 -0.55714286 -0.54285714 -0.52857143 -0.51428571 -0.5 -0.48571429 -0.47142857 -0.45714286 -0.44285714 -0.42857143 -0.41428571 -0.4 -0.38571429 -0.37142857 -0.35714286 -0.34285714 -0.32857143 -0.31428571 -0.3 -0.28571429 -0.27142857 -0.25714286 -0.24285714 -0.22857143 -0.21428571 -0.2 -0.18571429 -0.17142857 -0.15714286 -0.14285714 -0.12857143 -0.11428571 -0.1 -0.08571429 -0.07142857 -0.05714286 -0.04285714 -0.02857143 -0.01428571 0 0 0 0 0 0
  line L9 (-2.0572, -9.169) -> (-2.0111, -8.9635)
  arc A19 (-1.6061, -8.6959) -> (-2.0111, -8.9635) centre (-1.6696, -9.0401) ccw
  arc A20 (-1.6061, -8.6959) -> (-1.1597, -8.7666) centre (0, 0) ccw
  arc A21 (-0.8572, -9.1463) -> (-1.1597, -8.7666) centre (-1.2056, -9.1136) ccw
  line L10 (-0.8572, -9.1463) -> (-0.8768, -9.3559)
  spline S10 degree 5 poles (-0.8768, -9.3559) (-0.8772, -9.3606) (-0.878, -9.3699) (-0.8788, -9.3839) (-0.8791, -9.4026) (-0.8785, -9.426) (-0.8772, -9.4495) (-0.8755, -9.473) (-0.8735, -9.4965) (-0.8714, -9.52) (-0.8691, -9.5435) (-0.8666, -9.567) (-0.8638, -9.5906) (-0.8607, -9.6142) (-0.8572, -9.6377) (-0.8535, -9.6613) (-0.8494, -9.6849) (-0.8451, -9.7085) (-0.8406, -9.7321) (-0.836, -9.7557) (-0.8311, -9.7793) (-0.8261, -9.8029) (-0.8208, -9.8265) (-0.8153, -9.8501) (-0.8096, -9.8737) (-0.8037, -9.8973) (-0.7977, -9.9209) (-0.7914, -9.9445) (-0.7849, -9.968) (-0.7783, -9.9916) (-0.7715, -10.0152) (-0.7645, -10.0388) (-0.7574, -10.0623) (-0.7501, -10.0859) (-0.7426, -10.1095) (-0.7349, -10.133) (-0.7271, -10.1565) (-0.7191, -10.1801) (-0.711, -10.2036) (-0.7027, -10.2271) (-0.6942, -10.2506) (-0.6856, -10.2741) (-0.6768, -10.2976) (-0.6679, -10.321) (-0.6588, -10.3445) (-0.6496, -10.3679) (-0.6402, -10.3913) (-0.6307, -10.4148) (-0.621, -10.4382) (-0.6112, -10.4615) (-0.6013, -10.4849) (-0.5912, -10.5083) (-0.5809, -10.5316) (-0.5705, -10.5549) (-0.56, -10.5782) (-0.5493, -10.6015) (-0.5385, -10.6248) (-0.5276, -10.6481) (-0.5165, -10.6713) (-0.5053, -10.6945) (-0.4939, -10.7177) (-0.4824, -10.7409) (-0.4708, -10.7641) (-0.4591, -10.7872) (-0.4472, -10.8103) (-0.4352, -10.8334) (-0.423, -10.8565) (-0.4107, -10.8796) (-0.3983, -10.9026) (-0.3858, -10.9256) (-0.3731, -10.9486) (-0.3629, -10.967) (-0.3552, -10.9807) (-0.35, -10.9899) (-0.3474, -10.9945) knots 0 0 0 0 0 0 0.01428571 0.02857143 0.04285714 0.05714286 0.07142857 0.08571429 0.1 0.11428571 0.12857143 0.14285714 0.15714286 0.17142857 0.18571429 0.2 0.21428571 0.22857143 0.24285714 0.25714286 0.27142857 0.28571429 0.3 0.31428571 0.32857143 0.34285714 0.35714286 0.37142857 0.38571429 0.4 0.41428571 0.42857143 0.44285714 0.45714286 0.47142857 0.48571429 0.5 0.51428571 0.52857143 0.54285714 0.55714286 0.57142857 0.58571429 0.6 0.61428571 0.62857143 0.64285714 0.65714286 0.67142857 0.68571429 0.7 0.71428571 0.72857143 0.74285714 0.75714286 0.77142857 0.78571429 0.8 0.81428571 0.82857143 0.84285714 0.85714286 0.87142857 0.88571429 0.9 0.91428571 0.92857143 0.94285714 0.95714286 0.97142857 0.98571429 1 1 1 1 1 1
  arc A22 (-0.3474, -10.9945) -> (0.3474, -10.9945) centre (0, 0) ccw
  spline S11 degree 5 poles (0.3474, -10.9945) (0.35, -10.9899) (0.3552, -10.9807) (0.3629, -10.967) (0.3731, -10.9486) (0.3858, -10.9256) (0.3983, -10.9026) (0.4107, -10.8796) (0.423, -10.8565) (0.4352, -10.8334) (0.4472, -10.8103) (0.4591, -10.7872) (0.4708, -10.7641) (0.4824, -10.7409) (0.4939, -10.7177) (0.5053, -10.6945) (0.5165, -10.6713) (0.5276, -10.6481) (0.5385, -10.6248) (0.5493, -10.6015) (0.56, -10.5782) (0.5705, -10.5549) (0.5809, -10.5316) (0.5912, -10.5083) (0.6013, -10.4849) (0.6112, -10.4615) (0.621, -10.4382) (0.6307, -10.4148) (0.6402, -10.3913) (0.6496, -10.3679) (0.6588, -10.3445) (0.6679, -10.321) (0.6768, -10.2976) (0.6856, -10.2741) (0.6942, -10.2506) (0.7027, -10.2271) (0.711, -10.2036) (0.7191, -10.1801) (0.7271, -10.1565) (0.7349, -10.133) (0.7426, -10.1095) (0.7501, -10.0859) (0.7574, -10.0623) (0.7645, -10.0388) (0.7715, -10.0152) (0.7783, -9.9916) (0.7849, -9.968) (0.7914, -9.9445) (0.7977, -9.9209) (0.8037, -9.8973) (0.8096, -9.8737) (0.8153, -9.8501) (0.8208, -9.8265) (0.8261, -9.8029) (0.8311, -9.7793) (0.836, -9.7557) (0.8406, -9.7321) (0.8451, -9.7085) (0.8494, -9.6849) (0.8535, -9.6613) (0.8572, -9.6377) (0.8607, -9.6142) (0.8638, -9.5906) (0.8666, -9.567) (0.8691, -9.5435) (0.8714, -9.52) (0.8735, -9.4965) (0.8755, -9.473) (0.8772, -9.4495) (0.8785, -9.426) (0.8791, -9.4026) (0.8788, -9.3839) (0.878, -9.3699) (0.8772, -9.3606) (0.8768, -9.3559) knots -1 -1 -1 -1 -1 -1 -0.98571429 -0.97142857 -0.95714286 -0.94285714 -0.92857143 -0.91428571 -0.9 -0.88571429 -0.87142857 -0.85714286 -0.84285714 -0.82857143 -0.81428571 -0.8 -0.78571429 -0.77142857 -0.75714286 -0.74285714 -0.72857143 -0.71428571 -0.7 -0.68571429 -0.67142857 -0.65714286 -0.64285714 -0.62857143 -0.61428571 -0.6 -0.58571429 -0.57142857 -0.55714286 -0.54285714 -0.52857143 -0.51428571 -0.5 -0.48571429 -0.47142857 -0.45714286 -0.44285714 -0.42857143 -0.41428571 -0.4 -0.38571429 -0.37142857 -0.35714286 -0.34285714 -0.32857143 -0.31428571 -0.3 -0.28571429 -0.27142857 -0.25714286 -0.24285714 -0.22857143 -0.21428571 -0.2 -0.18571429 -0.17142857 -0.15714286 -0.14285714 -0.12857143 -0.11428571 -0.1 -0.08571429 -0.07142857 -0.05714286 -0.04285714 -0.02857143 -0.01428571 0 0 0 0 0 0
  line L11 (0.8768, -9.3559) -> (0.8572, -9.1463)
  arc A23 (1.1597, -8.7666) -> (0.8572, -9.1463) centre (1.2056, -9.1136) ccw
  arc A24 (1.1597, -8.7666) -> (1.6061, -8.6959) centre (0, 0) ccw
  arc A25 (2.0111, -8.9635) -> (1.6061, -8.6959) centre (1.6696, -9.0401) ccw
  line L12 (2.0111, -8.9635) -> (2.0572, -9.169)
  spline S12 degree 5 poles (2.0572, -9.169) (2.0583, -9.1735) (2.0604, -9.1826) (2.064, -9.1962) (2.0695, -9.2141) (2.0773, -9.2361) (2.0858, -9.2581) (2.0947, -9.2799) (2.1038, -9.3016) (2.1131, -9.3233) (2.1225, -9.345) (2.1322, -9.3666) (2.1421, -9.3881) (2.1524, -9.4096) (2.1629, -9.4309) (2.1738, -9.4522) (2.185, -9.4734) (2.1963, -9.4945) (2.2079, -9.5155) (2.2196, -9.5365) (2.2315, -9.5575) (2.2436, -9.5784) (2.2559, -9.5992) (2.2684, -9.6199) (2.2811, -9.6406) (2.294, -9.6612) (2.3071, -9.6818) (2.3204, -9.7023) (2.3338, -9.7227) (2.3474, -9.7431) (2.3611, -9.7634) (2.375, -9.7837) (2.3891, -9.8039) (2.4033, -9.8241) (2.4177, -9.8441) (2.4323, -9.8642) (2.447, -9.8841) (2.4619, -9.904) (2.4769, -9.9239) (2.492, -9.9437) (2.5074, -9.9634) (2.5228, -9.9831) (2.5384, -10.0027) (2.5541, -10.0223) (2.57, -10.0418) (2.586, -10.0612) (2.6022, -10.0806) (2.6185, -10.0999) (2.6349, -10.1192) (2.6515, -10.1384) (2.6682, -10.1575) (2.685, -10.1766) (2.702, -10.1957) (2.719, -10.2146) (2.7363, -10.2335) (2.7536, -10.2524) (2.7711, -10.2712) (2.7887, -10.2899) (2.8064, -10.3086) (2.8242, -10.3272) (2.8422, -10.3458) (2.8603, -10.3643) (2.8785, -10.3827) (2.8968, -10.4011) (2.9153, -10.4194) (2.9339, -10.4377) (2.9525, -10.4559) (2.9713, -10.474) (2.9903, -10.4921) (3.0093, -10.5101) (3.0284, -10.528) (3.0439, -10.5424) (3.0555, -10.5531) (3.0632, -10.5602) (3.0671, -10.5638) knots 0 0 0 0 0 0 0.01428571 0.02857143 0.04285714 0.05714286 0.07142857 0.08571429 0.1 0.11428571 0.12857143 0.14285714 0.15714286 0.17142857 0.18571429 0.2 0.21428571 0.22857143 0.24285714 0.25714286 0.27142857 0.28571429 0.3 0.31428571 0.32857143 0.34285714 0.35714286 0.37142857 0.38571429 0.4 0.41428571 0.42857143 0.44285714 0.45714286 0.47142857 0.48571429 0.5 0.51428571 0.52857143 0.54285714 0.55714286 0.57142857 0.58571429 0.6 0.61428571 0.62857143 0.64285714 0.65714286 0.67142857 0.68571429 0.7 0.71428571 0.72857143 0.74285714 0.75714286 0.77142857 0.78571429 0.8 0.81428571 0.82857143 0.84285714 0.85714286 0.87142857 0.88571429 0.9 0.91428571 0.92857143 0.94285714 0.95714286 0.97142857 0.98571429 1 1 1 1 1 1
  arc A26 (3.0671, -10.5638) -> (3.7279, -10.3491) centre (0, 0) ccw
  spline S13 degree 5 poles (3.7279, -10.3491) (3.7289, -10.3439) (3.731, -10.3336) (3.7341, -10.3181) (3.7382, -10.2974) (3.7431, -10.2717) (3.7479, -10.2459) (3.7526, -10.2202) (3.7572, -10.1944) (3.7616, -10.1687) (3.7659, -10.143) (3.77, -10.1174) (3.774, -10.0917) (3.7779, -10.0661) (3.7817, -10.0405) (3.7853, -10.0149) (3.7888, -9.9894) (3.7922, -9.9639) (3.7954, -9.9384) (3.7985, -9.9129) (3.8014, -9.8875) (3.8043, -9.862) (3.8069, -9.8366) (3.8095, -9.8113) (3.8119, -9.7859) (3.8141, -9.7606) (3.8162, -9.7354) (3.8182, -9.7101) (3.82, -9.6849) (3.8217, -9.6597) (3.8232, -9.6346) (3.8246, -9.6095) (3.8258, -9.5844) (3.8269, -9.5594) (3.8279, -9.5344) (3.8286, -9.5094) (3.8293, -9.4845) (3.8298, -9.4596) (3.8301, -9.4347) (3.8302, -9.4099) (3.8302, -9.3852) (3.8301, -9.3605) (3.8298, -9.3358) (3.8293, -9.3112) (3.8286, -9.2866) (3.8278, -9.2621) (3.8268, -9.2376) (3.8257, -9.2132) (3.8243, -9.1888) (3.8228, -9.1645) (3.8211, -9.1402) (3.8193, -9.116) (3.8172, -9.0919) (3.8149, -9.0678) (3.8124, -9.0438) (3.8097, -9.0199) (3.8069, -8.996) (3.8038, -8.9722) (3.8006, -8.9484) (3.7972, -8.9247) (3.7935, -8.9011) (3.7895, -8.8776) (3.7852, -8.8543) (3.7806, -8.831) (3.7757, -8.8078) (3.7706, -8.7848) (3.7653, -8.7617) (3.7599, -8.7388) (3.7543, -8.7159) (3.7483, -8.6932) (3.7416, -8.6708) (3.7355, -8.6531) (3.7305, -8.64) (3.7269, -8.6314) (3.725, -8.6271) knots -1 -1 -1 -1 -1 -1 -0.98571429 -0.97142857 -0.95714286 -0.94285714 -0.92857143 -0.91428571 -0.9 -0.88571429 -0.87142857 -0.85714286 -0.84285714 -0.82857143 -0.81428571 -0.8 -0.78571429 -0.77142857 -0.75714286 -0.74285714 -0.72857143 -0.71428571 -0.7 -0.68571429 -0.67142857 -0.65714286 -0.64285714 -0.62857143 -0.61428571 -0.6 -0.58571429 -0.57142857 -0.55714286 -0.54285714 -0.52857143 -0.51428571 -0.5 -0.48571429 -0.47142857 -0.45714286 -0.44285714 -0.42857143 -0.41428571 -0.4 -0.38571429 -0.37142857 -0.35714286 -0.34285714 -0.32857143 -0.31428571 -0.3 -0.28571429 -0.27142857 -0.25714286 -0.24285714 -0.22857143 -0.21428571 -0.2 -0.18571429 -0.17142857 -0.15714286 -0.14285714 -0.12857143 -0.11428571 -0.1 -0.08571429 -0.07142857 -0.05714286 -0.04285714 -0.02857143 -0.01428571 0 0 0 0 0 0
  line L13 (3.725, -8.6271) -> (3.6416, -8.4337)
  arc A27 (3.812, -7.9792) -> (3.6416, -8.4337) centre (3.9629, -8.295) ccw
  arc A28 (3.812, -7.9792) -> (4.2146, -7.774) centre (0, 0) ccw
  arc A29 (4.6826, -7.9033) -> (4.2146, -7.774) centre (4.3815, -8.0817) ccw
  line L14 (4.6826, -7.9033) -> (4.7899, -8.0845)
  spline S14 degree 5 poles (4.7899, -8.0845) (4.7923, -8.0885) (4.7972, -8.0965) (4.8048, -8.1083) (4.8155, -8.1236) (4.8298, -8.1422) (4.8446, -8.1604) (4.8598, -8.1784) (4.8752, -8.1962) (4.8907, -8.214) (4.9064, -8.2317) (4.9223, -8.2493) (4.9384, -8.2667) (4.9547, -8.2839) (4.9714, -8.301) (4.9883, -8.3178) (5.0055, -8.3345) (5.0228, -8.3511) (5.0403, -8.3675) (5.0579, -8.3839) (5.0757, -8.4001) (5.0937, -8.4162) (5.1118, -8.4322) (5.1301, -8.4481) (5.1486, -8.4639) (5.1672, -8.4795) (5.186, -8.495) (5.205, -8.5104) (5.224, -8.5257) (5.2433, -8.5409) (5.2626, -8.556) (5.2821, -8.5709) (5.3017, -8.5858) (5.3215, -8.6006) (5.3414, -8.6152) (5.3614, -8.6298) (5.3816, -8.6442) (5.4019, -8.6585) (5.4223, -8.6728) (5.4428, -8.6869) (5.4635, -8.701) (5.4843, -8.7149) (5.5052, -8.7287) (5.5262, -8.7425) (5.5473, -8.7561) (5.5686, -8.7697) (5.5899, -8.7831) (5.6114, -8.7964) (5.633, -8.8097) (5.6546, -8.8228) (5.6764, -8.8359) (5.6983, -8.8488) (5.7204, -8.8617) (5.7425, -8.8745) (5.7647, -8.8871) (5.787, -8.8997) (5.8094, -8.9122) (5.832, -8.9246) (5.8546, -8.9368) (5.8773, -8.949) (5.9001, -8.9611) (5.923, -8.9731) (5.9461, -8.985) (5.9692, -8.9969) (5.9924, -9.0086) (6.0157, -9.0202) (6.0391, -9.0317) (6.0626, -9.0432) (6.0861, -9.0545) (6.1098, -9.0658) (6.1336, -9.0769) (6.1526, -9.0858) (6.167, -9.0924) (6.1766, -9.0967) (6.1814, -9.0989) knots 0 0 0 0 0 0 0.01428571 0.02857143 0.04285714 0.05714286 0.07142857 0.08571429 0.1 0.11428571 0.12857143 0.14285714 0.15714286 0.17142857 0.18571429 0.2 0.21428571 0.22857143 0.24285714 0.25714286 0.27142857 0.28571429 0.3 0.31428571 0.32857143 0.34285714 0.35714286 0.37142857 0.38571429 0.4 0.41428571 0.42857143 0.44285714 0.45714286 0.47142857 0.48571429 0.5 0.51428571 0.52857143 0.54285714 0.55714286 0.57142857 0.58571429 0.6 0.61428571 0.62857143 0.64285714 0.65714286 0.67142857 0.68571429 0.7 0.71428571 0.72857143 0.74285714 0.75714286 0.77142857 0.78571429 0.8 0.81428571 0.82857143 0.84285714 0.85714286 0.87142857 0.88571429 0.9 0.91428571 0.92857143 0.94285714 0.95714286 0.97142857 0.98571429 1 1 1 1 1 1
  arc A30 (6.1814, -9.0989) -> (6.7435, -8.6906) centre (0, 0) ccw
  spline S15 degree 5 poles (6.7435, -8.6906) (6.7429, -8.6853) (6.7417, -8.6749) (6.7398, -8.6592) (6.7373, -8.6383) (6.734, -8.6122) (6.7306, -8.5863) (6.7271, -8.5603) (6.7235, -8.5345) (6.7198, -8.5086) (6.7159, -8.4829) (6.7119, -8.4572) (6.7079, -8.4316) (6.7036, -8.406) (6.6993, -8.3805) (6.6949, -8.355) (6.6903, -8.3297) (6.6856, -8.3044) (6.6808, -8.2791) (6.6758, -8.2539) (6.6708, -8.2288) (6.6656, -8.2038) (6.6603, -8.1788) (6.6549, -8.1539) (6.6493, -8.1291) (6.6436, -8.1043) (6.6378, -8.0796) (6.6319, -8.055) (6.6258, -8.0304) (6.6197, -8.006) (6.6133, -7.9816) (6.6069, -7.9573) (6.6003, -7.9331) (6.5936, -7.9089) (6.5868, -7.8848) (6.5798, -7.8609) (6.5727, -7.837) (6.5655, -7.8131) (6.5581, -7.7894) (6.5506, -7.7658) (6.543, -7.7422) (6.5352, -7.7188) (6.5273, -7.6954) (6.5192, -7.6722) (6.511, -7.649) (6.5026, -7.6259) (6.4941, -7.6029) (6.4855, -7.5801) (6.4767, -7.5573) (6.4677, -7.5346) (6.4586, -7.5121) (6.4493, -7.4897) (6.4399, -7.4673) (6.4303, -7.4452) (6.4205, -7.4231) (6.4106, -7.4011) (6.4005, -7.3793) (6.3902, -7.3576) (6.3798, -7.336) (6.3692, -7.3145) (6.3584, -7.2932) (6.3474, -7.2721) (6.3361, -7.2512) (6.3245, -7.2305) (6.3126, -7.21) (6.3007, -7.1896) (6.2886, -7.1694) (6.2763, -7.1492) (6.2639, -7.1292) (6.2512, -7.1095) (6.2379, -7.0902) (6.2267, -7.0752) (6.2178, -7.0643) (6.2117, -7.0572) (6.2086, -7.0537) knots -1 -1 -1 -1 -1 -1 -0.98571429 -0.97142857 -0.95714286 -0.94285714 -0.92857143 -0.91428571 -0.9 -0.88571429 -0.87142857 -0.85714286 -0.84285714 -0.82857143 -0.81428571 -0.8 -0.78571429 -0.77142857 -0.75714286 -0.74285714 -0.72857143 -0.71428571 -0.7 -0.68571429 -0.67142857 -0.65714286 -0.64285714 -0.62857143 -0.61428571 -0.6 -0.58571429 -0.57142857 -0.55714286 -0.54285714 -0.52857143 -0.51428571 -0.5 -0.48571429 -0.47142857 -0.45714286 -0.44285714 -0.42857143 -0.41428571 -0.4 -0.38571429 -0.37142857 -0.35714286 -0.34285714 -0.32857143 -0.31428571 -0.3 -0.28571429 -0.27142857 -0.25714286 -0.24285714 -0.22857143 -0.21428571 -0.2 -0.18571429 -0.17142857 -0.15714286 -0.14285714 -0.12857143 -0.11428571 -0.1 -0.08571429 -0.07142857 -0.05714286 -0.04285714 -0.02857143 -0.01428571 0 0 0 0 0 0
  line L15 (6.2086, -7.0537) -> (6.0695, -6.8957)
  arc A31 (6.0911, -6.4107) -> (6.0695, -6.8957) centre (6.3322, -6.6644) ccw
  arc A32 (6.0911, -6.4107) -> (6.4107, -6.0911) centre (0, 0) ccw
  arc A33 (6.8957, -6.0695) -> (6.4107, -6.0911) centre (6.6644, -6.3322) ccw
  line L16 (6.8957, -6.0695) -> (7.0537, -6.2086)
  spline S16 degree 5 poles (7.0537, -6.2086) (7.0572, -6.2117) (7.0643, -6.2178) (7.0752, -6.2267) (7.0902, -6.2379) (7.1095, -6.2512) (7.1292, -6.2639) (7.1492, -6.2763) (7.1694, -6.2886) (7.1896, -6.3007) (7.21, -6.3126) (7.2305, -6.3245) (7.2512, -6.3361) (7.2721, -6.3474) (7.2932, -6.3584) (7.3145, -6.3692) (7.336, -6.3798) (7.3576, -6.3902) (7.3793, -6.4005) (7.4011, -6.4106) (7.4231, -6.4205) (7.4452, -6.4303) (7.4673, -6.4399) (7.4897, -6.4493) (7.5121, -6.4586) (7.5346, -6.4677) (7.5573, -6.4767) (7.5801, -6.4855) (7.6029, -6.4941) (7.6259, -6.5026) (7.649, -6.511) (7.6722, -6.5192) (7.6954, -6.5273) (7.7188, -6.5352) (7.7422, -6.543) (7.7658, -6.5506) (7.7894, -6.5581) (7.8131, -6.5655) (7.837, -6.5727) (7.8609, -6.5798) (7.8848, -6.5868) (7.9089, -6.5936) (7.9331, -6.6003) (7.9573, -6.6069) (7.9816, -6.6133) (8.006, -6.6197) (8.0304, -6.6258) (8.055, -6.6319) (8.0796, -6.6378) (8.1043, -6.6436) (8.1291, -6.6493) (8.1539, -6.6549) (8.1788, -6.6603) (8.2038, -6.6656) (8.2288, -6.6708) (8.2539, -6.6758) (8.2791, -6.6808) (8.3044, -6.6856) (8.3297, -6.6903) (8.355, -6.6949) (8.3805, -6.6993) (8.406, -6.7036) (8.4316, -6.7079) (8.4572, -6.7119) (8.4829, -6.7159) (8.5086, -6.7198) (8.5345, -6.7235) (8.5603, -6.7271) (8.5863, -6.7306) (8.6122, -6.734) (8.6383, -6.7373) (8.6592, -6.7398) (8.6749, -6.7417) (8.6853, -6.7429) (8.6906, -6.7435) knots 0 0 0 0 0 0 0.01428571 0.02857143 0.04285714 0.05714286 0.07142857 0.08571429 0.1 0.11428571 0.12857143 0.14285714 0.15714286 0.17142857 0.18571429 0.2 0.21428571 0.22857143 0.24285714 0.25714286 0.27142857 0.28571429 0.3 0.31428571 0.32857143 0.34285714 0.35714286 0.37142857 0.38571429 0.4 0.41428571 0.42857143 0.44285714 0.45714286 0.47142857 0.48571429 0.5 0.51428571 0.52857143 0.54285714 0.55714286 0.57142857 0.58571429 0.6 0.61428571 0.62857143 0.64285714 0.65714286 0.67142857 0.68571429 0.7 0.71428571 0.72857143 0.74285714 0.75714286 0.77142857 0.78571429 0.8 0.81428571 0.82857143 0.84285714 0.85714286 0.87142857 0.88571429 0.9 0.91428571 0.92857143 0.94285714 0.95714286 0.97142857 0.98571429 1 1 1 1 1 1
  arc A34 (8.6906, -6.7435) -> (9.0989, -6.1814) centre (0, 0) ccw
  spline S17 degree 5 poles (9.0989, -6.1814) (9.0967, -6.1766) (9.0924, -6.167) (9.0858, -6.1526) (9.0769, -6.1336) (9.0658, -6.1098) (9.0545, -6.0861) (9.0432, -6.0626) (9.0317, -6.0391) (9.0202, -6.0157) (9.0086, -5.9924) (8.9969, -5.9692) (8.985, -5.9461) (8.9731, -5.923) (8.9611, -5.9001) (8.949, -5.8773) (8.9368, -5.8546) (8.9246, -5.832) (8.9122, -5.8094) (8.8997, -5.787) (8.8871, -5.7647) (8.8745, -5.7425) (8.8617, -5.7204) (8.8488, -5.6983) (8.8359, -5.6764) (8.8228, -5.6546) (8.8097, -5.633) (8.7964, -5.6114) (8.7831, -5.5899) (8.7697, -5.5686) (8.7561, -5.5473) (8.7425, -5.5262) (8.7287, -5.5052) (8.7149, -5.4843) (8.701, -5.4635) (8.6869, -5.4428) (8.6728, -5.4223) (8.6585, -5.4019) (8.6442, -5.3816) (8.6298, -5.3614) (8.6152, -5.3414) (8.6006, -5.3215) (8.5858, -5.3017) (8.5709, -5.2821) (8.556, -5.2626) (8.5409, -5.2433) (8.5257, -5.224) (8.5104, -5.205) (8.495, -5.186) (8.4795, -5.1672) (8.4639, -5.1486) (8.4481, -5.1301) (8.4322, -5.1118) (8.4162, -5.0937) (8.4001, -5.0757) (8.3839, -5.0579) (8.3675, -5.0403) (8.3511, -5.0228) (8.3345, -5.0055) (8.3178, -4.9883) (8.301, -4.9714) (8.2839, -4.9547) (8.2667, -4.9384) (8.2493, -4.9223) (8.2317, -4.9064) (8.214, -4.8907) (8.1962, -4.8752) (8.1784, -4.8598) (8.1604, -4.8446) (8.1422, -4.8298) (8.1236, -4.8155) (8.1083, -4.8048) (8.0965, -4.7972) (8.0885, -4.7923) (8.0845, -4.7899) knots -1 -1 -1 -1 -1 -1 -0.98571429 -0.97142857 -0.95714286 -0.94285714 -0.92857143 -0.91428571 -0.9 -0.88571429 -0.87142857 -0.85714286 -0.84285714 -0.82857143 -0.81428571 -0.8 -0.78571429 -0.77142857 -0.75714286 -0.74285714 -0.72857143 -0.71428571 -0.7 -0.68571429 -0.67142857 -0.65714286 -0.64285714 -0.62857143 -0.61428571 -0.6 -0.58571429 -0.57142857 -0.55714286 -0.54285714 -0.52857143 -0.51428571 -0.5 -0.48571429 -0.47142857 -0.45714286 -0.44285714 -0.42857143 -0.41428571 -0.4 -0.38571429 -0.37142857 -0.35714286 -0.34285714 -0.32857143 -0.31428571 -0.3 -0.28571429 -0.27142857 -0.25714286 -0.24285714 -0.22857143 -0.21428571 -0.2 -0.18571429 -0.17142857 -0.15714286 -0.14285714 -0.12857143 -0.11428571 -0.1 -0.08571429 -0.07142857 -0.05714286 -0.04285714 -0.02857143 -0.01428571 0 0 0 0 0 0
  line L17 (8.0845, -4.7899) -> (7.9033, -4.6826)
  arc A35 (7.774, -4.2146) -> (7.9033, -4.6826) centre (8.0817, -4.3815) ccw
  arc A36 (7.774, -4.2146) -> (7.9792, -3.812) centre (0, 0) ccw
  arc A37 (8.4337, -3.6416) -> (7.9792, -3.812) centre (8.295, -3.9629) ccw
  line L18 (8.4337, -3.6416) -> (8.6271, -3.725)